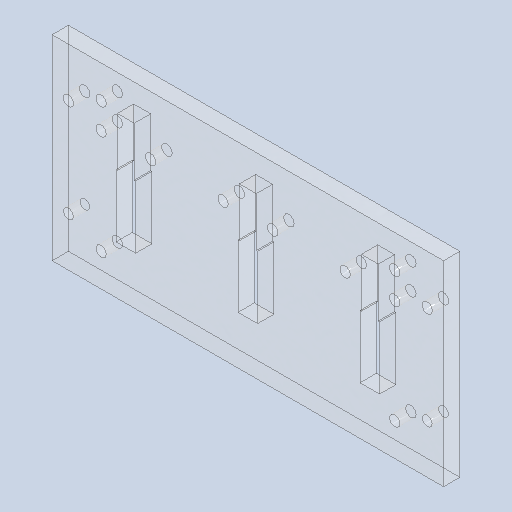
# Autodesk Inventor part: part1
Saved by Autodesk Inventor 2025.2 (Build 292293000, 293)
## iProperties
Created: 2025-02-28
Part Number: part1
Material: アクリル、クリア
Document SubType Name: Modeling
Designer: haruy
Density: 1.19 g/cm^3
Appearance: 透明 - クリア
Author: haruy
Autodesk Inventor part; units mm, degrees
ref_plane "YZ Plane" through (0, 0, 0) normal (1, 0, 0) x (0, 1, 0)
ref_plane "XZ Plane" through (0, 0, 0) normal (0, 1, 0) x (-1, 0, 0)
ref_plane "XY Plane" through (0, 0, 0) normal (0, 0, 1) x (1, 0, 0)
derived "oikon-Sketch-Base.ipt"
sketch "スケッチ1" plane through (100, 0, 0) normal (1, 0, 0) x (0, 1, 0)
  line L0 (0, 0) -> (-50, 0)
  line L1 (-50, 0) -> (-50, -5)
  line L2 (-50, -5) -> (0, -5)
  line L3 (0, -5) -> (0, 0)
  circle A0 centre (-9, -9) radius 4
  circle A1 centre (-9, -9) radius 7
  line L4 (-21, 5) -> (-40, 5)
  line L5 (-40, 5) -> (-40, -5)
  line L6 (-40, -5) -> (-21, -5)
  line L7 (-21, -5) -> (-21, 5)
  line L8 (0, 8.5) -> (-50, 8.5)
  line L9 (-50, 8.5) -> (-50, 7)
  line L10 (-50, 7) -> (0, 7)
  line L11 (0, 7) -> (0, 8.5)
  line L12 (0, 18.5) -> (-50, 18.5)
  line L13 (-50, 18.5) -> (-50, 13.5)
  line L14 (-50, 13.5) -> (0, 13.5)
  line L15 (0, 13.5) -> (0, 18.5)
  line L16 (-10.8313, -2.2438) -> (-39.7865, -10.092)
  arc A2 (-29, -5) -> (-27, -5) centre (-28, -5) ccw
  line L17 (-7.1687, -15.7562) -> (-36.124, -23.6045)
  line L18 (-39.7865, -10.092) -> (-36.124, -23.6045)
  line L19 (-36.124, -23.6045) -> (-30.8918, -42.908)
  arc A3 (-36.124, -23.6045) -> (-33.5079, -33.2562) centre (-34.8159, -28.4303) ccw
  line L20 (-33.5079, -33.2562) -> (-19.0303, -29.3321)
  line L21 (-19.0303, -29.3321) -> (-16.8241, -37.4713)
  arc A4 (-16.4142, -38.9838) -> (-19.0303, -29.3321) centre (-17.7222, -34.158) ccw
  line L22 (-16.4142, -38.9838) -> (-30.8918, -42.908)
  arc A5 (-39.7865, -10.092) -> (-30.8918, -42.908) centre (-35.3391, -26.5) ccw
  line L23 (0, 0) -> (5, 0)
  line L24 (5, 0) -> (5, -5)
  line L25 (5, -5) -> (0, -5)
  line L26 (0, -5) -> (0, 0)
  line L27 (0, 18.5) -> (5, 18.5)
  line L28 (5, 18.5) -> (5, 13.5)
  line L29 (5, 13.5) -> (0, 13.5)
  line L30 (0, 13.5) -> (0, 18.5)
  line L31 (-50, 18.5) -> (-55, 18.5)
  line L32 (-55, 18.5) -> (-55, 13.5)
  line L33 (-55, 13.5) -> (-50, 13.5)
  line L34 (-50, 13.5) -> (-50, 18.5)
  line L35 (-50, 0) -> (-55, 0)
  line L36 (-55, 0) -> (-55, -5)
  line L37 (-55, -5) -> (-50, -5)
  line L38 (-50, -5) -> (-50, 0)
  point P0 (-14.1989, -5)
sketch "スケッチ2" plane through (0, 0, 0) normal (0, 0, 1) x (1, 0, 0)
  line L0 (0, 0) -> (-100, 0)
  line L1 (-100, 0) -> (-100, -50)
  line L2 (-100, -50) -> (0, -50)
  line L3 (0, -50) -> (0, 0)
  line L4 (0, -9) -> (-25.2, -9)
  line L5 (-25.2, -9) -> (-25.2, -17)
  line L6 (-25.2, -17) -> (0, -17)
  line L7 (0, -17) -> (0, -9)
  line L8 (0, -50) -> (10, -50)
  line L9 (10, -50) -> (10, 0)
  line L10 (10, 0) -> (0, 0)
  line L11 (0, 0) -> (0, -50)
  line L12 (-100, -50) -> (-110, -50)
  line L13 (-110, -50) -> (-110, 0)
  line L14 (-110, 0) -> (-100, 0)
  line L15 (-100, 0) -> (-100, -50)
  line L16 (-10.1, -6) -> (-15.1, -6)
  line L17 (-15.1, -6) -> (-15.1, -20.9)
  line L18 (-15.1, -20.9) -> (-10.1, -20.9)
  line L19 (-10.1, -20.9) -> (-10.1, -6)
  circle A0 centre (-5, -13) radius 1.6
  line L20 (-12.6, -20.9) -> (-12.6, -6)
  circle A1 centre (-20.2, -13) radius 1.6
  line L21 (-37.4, -9) -> (-62.6, -9)
  line L22 (-62.6, -9) -> (-62.6, -17)
  line L23 (-62.6, -17) -> (-37.4, -17)
  line L24 (-37.4, -17) -> (-37.4, -9)
  circle A2 centre (-42.4, -13) radius 1.6
  circle A3 centre (-57.6, -13) radius 1.6
  circle A4 centre (-79.8, -13) radius 1.6
  circle A5 centre (-95, -13) radius 1.6
  circle A6 centre (5, -10) radius 1.6
  circle A7 centre (5, -40) radius 1.5
  line L25 (-50, 0) -> (-50, -50)
  circle A8 centre (-105, -10) radius 1.6
  circle A9 centre (-105, -40) radius 1.5
  line L26 (-47.5, -6) -> (-52.5, -6)
  line L27 (-52.5, -6) -> (-52.5, -40.2)
  line L28 (-52.5, -40.2) -> (-47.5, -40.2)
  line L29 (-47.5, -40.2) -> (-47.5, -6)
  line L30 (-84.9, -6) -> (-89.9, -6)
  line L31 (-89.9, -6) -> (-89.9, -35.3712)
  line L32 (-89.9, -35.3712) -> (-84.9, -35.3712)
  line L33 (-84.9, -35.3712) -> (-84.9, -6)
  line L34 (10, 0) -> (-110, 0)
  line L35 (-110, 0) -> (-110, 5)
  line L36 (-110, 5) -> (10, 5)
  line L37 (10, 5) -> (10, 0)
  line L38 (10, -50) -> (-110, -50)
  line L39 (-110, -50) -> (-110, -55)
  line L40 (-110, -55) -> (10, -55)
  line L41 (10, -55) -> (10, -50)
  circle A10 centre (-5, -5) radius 1.6
  line L42 (10, -25) -> (-100, -25)
  circle A11 centre (-5, -45) radius 1.6
  circle A12 centre (-95, -45) radius 1.6
  circle A13 centre (-95, -5) radius 1.6
  line L43 (-15.2, -5.9) -> (-10, -5.9)
  line L44 (-10, -5.9) -> (-10, -21)
  line L45 (-10, -21) -> (-15.2, -21)
  line L46 (-15.2, -21) -> (-15.2, -5.9)
  line L47 (-9.6, -40.2) -> (-15.6, -40.2)
  line L48 (-15.6, -40.2) -> (-15.6, -21)
  line L49 (-15.6, -21) -> (-9.6, -21)
  line L50 (-9.6, -21) -> (-9.6, -40.2)
  line L51 (-53, -40.2) -> (-53, -21)
  line L52 (-47, -40.2) -> (-53, -40.2)
  line L53 (-47, -21) -> (-47, -40.2)
  line L54 (-53, -21) -> (-47, -21)
  line L55 (-47.4, -5.9) -> (-47.4, -21)
  line L56 (-52.6, -21) -> (-52.6, -5.9)
  line L57 (-52.6, -5.9) -> (-47.4, -5.9)
  line L58 (-90.4, -40.2) -> (-90.4, -21)
  line L59 (-84.4, -40.2) -> (-90.4, -40.2)
  line L60 (-84.4, -21) -> (-84.4, -40.2)
  line L61 (-90.4, -21) -> (-84.4, -21)
  line L62 (-84.8, -5.9) -> (-84.8, -21)
  line L63 (-90, -21) -> (-90, -5.9)
  line L64 (-90, -5.9) -> (-84.8, -5.9)
ref_plane "作業平面1" through (100, 0, 0) normal (1, 0, 0) x (0, 1, 0)
extrude "押し出し1" add sketch "スケッチ2" along normal blind 5 contours L3 L4 L44 L43 L46 L5 L6 L49 L48 L42 L53 L54 L55 L23 L24 L21 L57 L25 L0 | L10 L9 L42 L3 | L0 L14 L35 L36 L37 L10 | L25 L57 L56 L21 L22 L23 L54 L51 L42 L60 L61 L62 L64 L63 L58 L1 L0 | L3 L6 L44 L4 | L1 L12 L13 L14 | L3 L42 L50 L49 L44 L6 | L9 L8 L3 L42 | L42 L58 L59 L60 L51 L52 L28 L25 L2 L1 | L3 L2 L25 L28 L52 L53 L42 L48 L47 L50 | L41 L40 L39 L12 L2 L8 | L56 L23 L22 L21 | L21 L24 L23 L55 | L46 L6 L5 L4
